Autodesk Inventor part; units mm, degrees
(part 15 of 18)
  ellipse E448 centre (-10.0711, -17.3808) end of major axis (-10.0127, -17.5616) minor radius 0.168 (-10.201, -17.4916) -> (-10.0699, -17.5684) ccw
  ellipse E449 centre (-10.0044, -17.3592) end of major axis (-9.946, -17.54) minor radius 0.168 (-10.1746, -17.347) -> (-10.0032, -17.5468) ccw
  ellipse E450 centre (-10.0405, -11.8092) end of major axis (-10.0989, -11.6284) minor radius 0.168 (-10.0418, -11.6216) -> (-10.2107, -11.797) ccw
  line L564 (-10.1657, -11.65) -> (-10.0989, -11.6284)
  line L565 (-10.0699, -17.5684) -> (-9.8829, -17.5818)
  line L566 (-9.6221, -17.6005) -> (-9.2494, -17.6273)
  line L567 (-10.1746, -17.347) -> (-10.1836, -15.9644)
  line L568 (-9.8264, -17.5595) -> (-10.0032, -17.5468)
  line L569 (-10.0418, -11.6216) -> (-9.5939, -11.6537)
  line L570 (-10.2017, -13.1796) -> (-10.2107, -11.797)
  ellipse E451 centre (-9.5952, -13.6245) end of major axis (-9.6536, -13.4437) minor radius 0.168 (-9.4538, -13.5315) -> (-9.5964, -13.4369) ccw
  ellipse E452 centre (-10.6816, -15.6958) end of major axis (-10.6952, -15.8853) minor radius 0.0836 (-10.7661, -15.7231) -> (-10.7542, -15.813) ccw
  ellipse E453 centre (-10.6948, -13.6615) end of major axis (-10.6812, -13.472) minor radius 0.0836 (-10.696, -13.4739) -> (-10.7106, -13.4814) ccw
  ellipse E454 centre (-10.6948, -13.6615) end of major axis (-10.7084, -13.851) minor radius 0.0836 (-10.7728, -13.6118) -> (-10.7793, -13.6888) ccw
  ellipse E455 centre (-9.5285, -13.603) end of major axis (-9.5869, -13.4222) minor radius 0.168 (-9.4742, -13.4296) -> (-9.5297, -13.4153) ccw
  ellipse E456 centre (-10.5472, -15.7055) end of major axis (-10.5336, -15.516) minor radius 0.0836 (-10.6318, -15.7328) -> (-10.626, -15.7965) ccw
  ellipse E457 centre (-10.5605, -13.6711) end of major axis (-10.5469, -13.4816) minor radius 0.0836 (-10.6385, -13.6213) -> (-10.645, -13.6984) ccw
  line L571 (-10.3369, -13.1699) -> (-10.3459, -11.7873)
  line L572 (-10.4317, -11.627) -> (-10.6574, -11.6999)
  line L573 (-10.7526, -17.6683) -> (-10.3931, -17.5522)
  line L574 (-10.3098, -17.3373) -> (-10.3188, -15.9547)
  line L575 (-10.2026, -13.1795) -> (-10.2116, -11.797)
  line L576 (-10.1755, -17.3469) -> (-10.1845, -15.9644)
  line L577 (-11.2285, -17.875) -> (-10.2588, -17.5619)
  ellipse E458 centre (-10.4305, -11.8146) end of major axis (-10.4169, -11.6251) minor radius 0.0836 (-10.3459, -11.7873) -> (-10.4317, -11.627) ccw
  ellipse E459 centre (-10.3943, -17.3646) end of major axis (-10.4079, -17.5541) minor radius 0.0836 (-10.3931, -17.5522) -> (-10.3098, -17.3373) ccw
  ellipse E460 centre (-10.2961, -11.8243) end of major axis (-10.2825, -11.6347) minor radius 0.0836 (-10.2116, -11.797) -> (-10.2825, -11.6347) ccw
  ellipse E461 centre (-10.26, -17.3742) end of major axis (-10.2736, -17.5637) minor radius 0.0836 (-10.2588, -17.5619) -> (-10.1755, -17.3469) ccw
  line L578 (-10.4169, -11.6251) -> (-10.2825, -11.6347)
  line L579 (-10.9931, -17.9358) -> (-11.1159, -17.927)
  line L580 (-11.1826, -17.9486) -> (-10.9615, -17.9644)
  ellipse E462 centre (-11.0046, -17.8911) end of major axis (-11.2546, -17.8927) minor radius 0.0393 (-11.2285, -17.875) -> (-11.1159, -17.927) ccw
  ellipse E463 centre (-11.0046, -17.8911) end of major axis (-10.6047, -17.8885) minor radius 0.0629 (-11.3596, -17.9224) -> (-11.1826, -17.9486) ccw
  line L581 (9.5691, -13.3926) -> (9.6692, -13.3931)
  line L582 (9.5609, -13.4102) -> (9.5315, -13.41)
  line L583 (9.6942, -15.6278) -> (9.4944, -13.5809)
  ellipse E464 centre (9.7188, -11.8144) end of major axis (9.6943, -11.6259) minor radius 0.0925 (9.7186, -11.6292) -> (9.7004, -11.6256) ccw
  ellipse E465 centre (10.134, -17.4154) end of major axis (10.1585, -17.6038) minor radius 0.0925 (10.1524, -17.6042) -> (10.1585, -17.6038) ccw
  line L584 (10.159, -17.6038) -> (10.1585, -17.6038)
  line L585 (9.7004, -11.6256) -> (9.6471, -11.6253)
  line L586 (9.7129, -17.5843) -> (10.0159, -17.5859)
  line L587 (9.531, -17.601) -> (9.9137, -17.603)
  line L588 (10.1514, -17.6042) -> (10.1524, -17.6042)
  ellipse E466 centre (9.7873, -15.6283) end of major axis (9.8118, -15.8167) minor radius 0.0925 (9.6942, -15.6278) -> (9.7563, -15.7911) ccw
  ellipse E467 centre (9.5875, -13.5814) end of major axis (9.563, -13.393) minor radius 0.0925 (9.5691, -13.3926) -> (9.4944, -13.5809) ccw
  line L589 (-9.3645, -11.6259) -> (-9.6015, -11.6308)
  line L590 (-9.9346, -17.5873) -> (-9.6926, -17.5823)
  line L591 (-9.8266, -17.6047) -> (-9.5717, -17.5995)
  line L592 (-9.6593, -13.3971) -> (-9.5198, -13.3942)
  line L593 (-9.4932, -13.9726) -> (-9.655, -15.6281)
  line L594 (-9.4847, -13.4131) -> (-9.5251, -13.4139)
  ellipse E468 centre (-9.5383, -13.583) end of major axis (-9.5146, -13.3945) minor radius 0.0827 (-9.4531, -13.5262) -> (-9.5198, -13.3942) ccw
  ellipse E469 centre (-9.7384, -15.6298) end of major axis (-9.7147, -15.4413) minor radius 0.0827 (-9.7169, -15.7972) -> (-9.655, -15.6281) ccw
  ellipse E470 centre (-9.2442, -11.6758) end of major axis (-9.6423, -11.6369) minor radius 0.023 (-9.6015, -11.6308) -> (-9.6423, -11.6369) ccw
  line L595 (-9.6423, -11.6369) -> (-9.6436, -11.6502)
  line L596 (11.1852, -17.9034) -> (11.022, -17.917)
  line L597 (11.0263, -17.9438) -> (11.2596, -17.9243)
  ellipse E471 centre (11.1864, -17.7157) end of major axis (11.1349, -17.8986) minor radius 0.1628 (11.1852, -17.9034) -> (11.2728, -17.8675) ccw
  ellipse E472 centre (11.2609, -17.7367) end of major axis (11.2094, -17.9196) minor radius 0.1628 (11.2596, -17.9243) -> (11.3195, -17.9066) ccw
  line L598 (10.4073, -13.401) -> (10.5863, -13.4514)
  line L599 (10.7882, -13.6963) -> (10.7746, -15.7306)
  ellipse E473 centre (10.0601, -13.43) end of major axis (10.4601, -13.4327) minor radius 0.0629 (10.4073, -13.401) -> (9.8616, -13.3741) ccw
  line L600 (9.6609, -13.3908) -> (9.8616, -13.3741)
  line L601 (9.936, -13.3951) -> (9.5169, -13.43)
  ellipse E474 centre (10.0601, -13.43) end of major axis (9.8101, -13.4283) minor radius 0.0393 (10.2771, -13.4119) -> (9.936, -13.3951) ccw
  line L602 (10.4387, -13.4574) -> (10.2771, -13.4119)
  line L603 (9.8455, -15.7837) -> (9.7306, -15.7933)
  ellipse E475 centre (10.044, -15.8396) end of major axis (9.644, -15.8369) minor radius 0.0629 (10.3509, -15.8012) -> (9.8455, -15.7837) ccw
  line L604 (10.6444, -15.7415) -> (10.6474, -15.29)
  line L605 (10.6548, -14.1819) -> (10.658, -13.7071)
  ellipse E476 centre (10.6939, -13.6697) end of major axis (10.6781, -13.4804) minor radius 0.0933 (10.7882, -13.6963) -> (10.7803, -13.6162) ccw
  ellipse E477 centre (10.6804, -15.704) end of major axis (10.6646, -15.5147) minor radius 0.0933 (10.7577, -15.8313) -> (10.7746, -15.7306) ccw
  ellipse E478 centre (10.5637, -13.6806) end of major axis (10.5795, -13.8699) minor radius 0.0933 (10.658, -13.7071) -> (10.6537, -13.6478) ccw
  ellipse E479 centre (10.5501, -15.7149) end of major axis (10.5659, -15.9042) minor radius 0.0933 (10.6441, -15.7534) -> (10.6444, -15.7415) ccw
  ellipse E480 centre (10.5501, -15.7149) end of major axis (10.5659, -15.9042) minor radius 0.0933 (10.6349, -15.8188) -> (10.6426, -15.7751) ccw
  line L606 (10.3796, -17.5684) -> (10.5328, -17.6116)
  line L607 (10.2493, -17.5793) -> (11.3312, -17.8839)
  line L608 (9.8733, -11.6163) -> (9.6559, -11.6344)
  ellipse E481 centre (10.0323, -17.5974) end of major axis (10.2823, -17.5991) minor radius 0.0393 (10.2493, -17.5793) -> (9.9154, -17.5619) ccw
  ellipse E482 centre (10.0718, -11.6722) end of major axis (9.6718, -11.6695) minor radius 0.0629 (10.3988, -11.6381) -> (9.8733, -11.6163) ccw
  ellipse E483 centre (10.0323, -17.5974) end of major axis (9.6323, -17.5947) minor radius 0.0629 (10.3796, -17.5684) -> (9.8379, -17.5412) ccw
  ellipse E484 centre (11.3324, -17.6963) end of major axis (11.3482, -17.8857) minor radius 0.0933 (11.3312, -17.8839) -> (11.3482, -17.8857) ccw
  line L609 (11.4013, -17.8812) -> (11.3482, -17.8857)
  ellipse E485 centre (-10.0243, -17.7521) end of major axis (-10.4666, -17.7632) minor radius 0.0741 (-10.1871, -17.6872) -> (-10.2508, -17.694) ccw
  ellipse E486 centre (-10.174, -17.7137) end of major axis (-10.0241, -17.7099) minor radius 0.0251 (-10.2508, -17.694) -> (-10.312, -17.7072) ccw
  ellipse E487 centre (-10.5584, -17.8746) end of major axis (-10.7084, -17.8783) minor radius 0.0251 (-10.6964, -17.8681) -> (-10.7083, -17.8774) ccw
  ellipse E488 centre (-10.5248, -17.8877) end of major axis (-10.6748, -17.8914) minor radius 0.0251 (-10.6523, -17.904) -> (-10.6494, -17.9047) ccw
  line L610 (-10.6964, -17.8681) -> (-10.6465, -17.8472)
  line L611 (-10.543, -17.8039) -> (-10.5099, -17.79)
  line L612 (-10.3387, -17.7184) -> (-10.312, -17.7072)
  line L613 (-9.0741, -17.7927) -> (-9.1333, -17.8175)
  ellipse E489 centre (-9.8556, -17.818) end of major axis (-9.2758, -17.8034) minor radius 0.0971 (-9.8744, -17.7214) -> (-10.3177, -17.7706) ccw
  ellipse E490 centre (-10.3496, -17.7345) end of major axis (-10.1998, -17.7269) minor radius 0.0268 (-10.3677, -17.7087) -> (-10.3792, -17.7096) ccw
  ellipse E491 centre (-10.3496, -17.7345) end of major axis (-10.1998, -17.7269) minor radius 0.0268 (-10.3138, -17.7067) -> (-10.3238, -17.7068) ccw
  ellipse E492 centre (-10.4338, -17.7442) end of major axis (-10.284, -17.7366) minor radius 0.0268 (-10.5065, -17.7242) -> (-10.5698, -17.7395) ccw
  ellipse E493 centre (-10.8456, -17.924) end of major axis (-10.9954, -17.9315) minor radius 0.0268 (-10.9816, -17.9194) -> (-10.9924, -17.9364) ccw
  ellipse E494 centre (-10.8146, -17.9375) end of major axis (-10.9644, -17.9451) minor radius 0.0268 (-10.9456, -17.957) -> (-10.8774, -17.965) ccw
  line L614 (-10.9961, -17.9176) -> (-10.9954, -17.9315)
  ellipse E495 centre (-10.292, -17.783) end of major axis (-10.734, -17.8053) minor radius 0.0791 (-10.3792, -17.7096) -> (-10.5065, -17.7242) ccw
  ellipse E496 centre (-10.5592, -17.8996) end of major axis (-11.0011, -17.922) minor radius 0.0791 (-10.9924, -17.9364) -> (-10.9456, -17.957) ccw
  line L615 (-10.9816, -17.9194) -> (-10.5698, -17.7395)
  line L616 (-10.646, -17.9728) -> (-10.8774, -17.965)
  ellipse E497 centre (-10.1365, -17.8511) end of major axis (-10.7157, -17.8804) minor radius 0.1037 (-10.1103, -17.7462) -> (-10.6484, -17.9247) ccw
  ellipse E498 centre (10.8498, -17.9277) end of major axis (10.7, -17.9201) minor radius 0.0268 (10.9264, -17.9545) -> (10.9876, -17.945) ccw
  ellipse E499 centre (10.872, -17.9132) end of major axis (11.0218, -17.9208) minor radius 0.0268 (11.0211, -17.9231) -> (11.0008, -17.9058) ccw
  ellipse E500 centre (10.3706, -17.7374) end of major axis (10.5204, -17.745) minor radius 0.0268 (10.4994, -17.73) -> (10.4295, -17.7156) ccw
  ellipse E501 centre (10.2837, -17.7292) end of major axis (10.4335, -17.7368) minor radius 0.0268 (10.2156, -17.7019) -> (10.2072, -17.7023) ccw
  line L617 (11.0218, -17.9208) -> (11.0227, -17.9032)
  ellipse E502 centre (10.5812, -17.894) end of major axis (11.0231, -17.9164) minor radius 0.0791 (10.9876, -17.945) -> (11.0211, -17.9231) ccw
  ellipse E503 centre (10.2559, -17.7799) end of major axis (9.814, -17.7575) minor radius 0.0791 (10.4295, -17.7156) -> (10.3776, -17.7098) ccw
  line L618 (10.4994, -17.73) -> (11.0008, -17.9058)
  line L619 (9.9244, -17.7186) -> (9.9274, -17.7184)
  line L620 (10.1429, -17.706) -> (10.2072, -17.7023)
  line L621 (10.9264, -17.9545) -> (10.6544, -17.9701)
  ellipse E504 centre (10.1447, -17.8527) end of major axis (10.724, -17.882) minor radius 0.1037 (10.6566, -17.9263) -> (10.1185, -17.7477) ccw
  line L622 (9.0199, -17.8982) -> (9.1408, -17.9388)
  ellipse E505 centre (8.5314, -18.0839) end of major axis (9.1087, -18.0281) minor radius 0.1485 (9.1077, -18.0416) -> (9.0262, -17.9624) ccw
  line L623 (-9.1325, -17.937) -> (-9.0106, -17.8853)
  ellipse E506 centre (-8.5232, -18.0826) end of major axis (-9.1005, -18.0268) minor radius 0.1485 (-9.018, -17.961) -> (-9.0995, -18.0402) ccw
  ellipse E507 centre (-9.8417, -17.6845) end of major axis (-9.6917, -17.6835) minor radius 0.0236 (-9.775, -17.663) -> (-9.8671, -17.6614) ccw
  ellipse E508 centre (-9.9269, -17.6896) end of major axis (-9.7769, -17.6886) minor radius 0.0236 (-9.9959, -17.6691) -> (-10.0612, -17.6799) ccw
  ellipse E509 centre (-9.7922, -17.7295) end of major axis (-10.2347, -17.7324) minor radius 0.0696 (-9.8671, -17.6614) -> (-9.9959, -17.6691) ccw
  line L624 (-10.131, -17.7025) -> (-10.0612, -17.6799)
  line L625 (-9.0059, -17.8375) -> (-9.1329, -17.8786)
  line L626 (-9.775, -17.663) -> (-8.9943, -17.719)
  ellipse E510 centre (-9.6485, -17.7958) end of major axis (-9.0685, -17.7921) minor radius 0.0912 (-9.1332, -17.8344) -> (-10.1349, -17.7493) ccw
  ellipse E511 centre (9.1837, -17.6745) end of major axis (9.0344, -17.6891) minor radius 0.0086 (9.3146, -17.666) -> (9.3198, -17.6649) ccw
  ellipse E512 centre (9.1837, -17.6745) end of major axis (9.0344, -17.6891) minor radius 0.0086 (9.2572, -17.6749) -> (9.2595, -17.6746) ccw
  ellipse E513 centre (9.2076, -17.6672) end of major axis (9.3569, -17.6526) minor radius 0.0086 (9.3559, -17.6538) -> (9.3375, -17.6503) ccw
  line L627 (9.3569, -17.6526) -> (9.3542, -17.6252)
  ellipse E514 centre (8.9184, -17.6934) end of major axis (9.3588, -17.6504) minor radius 0.0254 (9.3198, -17.6649) -> (9.3559, -17.6538) ccw
  line L628 (8.9449, -17.6482) -> (9.3375, -17.6503)
  line L629 (9.2572, -17.6749) -> (9.0014, -17.7082)
  ellipse E515 centre (8.4859, -17.7285) end of major axis (9.0632, -17.6721) minor radius 0.0333 (9, -17.6937) -> (8.9426, -17.6636) ccw
  line L630 (-9.3231, -17.6523) -> (-8.937, -17.6444)
  line L631 (-8.9932, -17.7076) -> (-9.2261, -17.6783)
  ellipse E516 centre (-9.1891, -17.6692) end of major axis (-9.3384, -17.6546) minor radius 0.0086 (-9.3231, -17.6523) -> (-9.3362, -17.6564) ccw
  ellipse E517 centre (-9.1603, -17.6769) end of major axis (-9.3096, -17.6623) minor radius 0.0086 (-9.2925, -17.6681) -> (-9.2261, -17.6783) ccw
  line L632 (-9.3367, -17.6373) -> (-9.3384, -17.6546)
  ellipse E518 centre (-8.9024, -17.6942) end of major axis (-9.3428, -17.6512) minor radius 0.0254 (-9.3362, -17.6564) -> (-9.2925, -17.6681) ccw
  ellipse E519 centre (-8.4777, -17.7272) end of major axis (-9.0549, -17.6708) minor radius 0.0333 (-8.9343, -17.6622) -> (-8.9917, -17.6924) ccw
  line L633 (10.0249, -17.6776) -> (10.2019, -17.7274)
  line L634 (10.3294, -17.7633) -> (10.3379, -17.7657)
  line L635 (9.0029, -17.7241) -> (9.7336, -17.6632)
  line L636 (9.1412, -17.8755) -> (9.0142, -17.8398)
  ellipse E520 centre (9.8946, -17.6884) end of major axis (10.0446, -17.6894) minor radius 0.0236 (10.0249, -17.6776) -> (9.9558, -17.6673) ccw
  ellipse E521 centre (9.808, -17.6842) end of major axis (9.958, -17.6852) minor radius 0.0236 (9.8248, -17.6608) -> (9.7336, -17.6632) ccw
  ellipse E522 centre (9.7753, -17.7297) end of major axis (9.3328, -17.7267) minor radius 0.0696 (9.9558, -17.6673) -> (9.8248, -17.6608) ccw
  ellipse E523 centre (9.6567, -17.7973) end of major axis (9.0767, -17.7934) minor radius 0.0912 (10.1432, -17.7508) -> (9.1414, -17.8358) ccw
  line L637 (-10.5777, -15.7864) -> (-10.6036, -15.7973)
  line L638 (-10.6449, -13.7102) -> (-10.63, -13.7039)
  line L639 (-10.5317, -15.7886) -> (-10.5563, -15.7989)
  line L640 (-10.5777, -15.7864) -> (-10.5802, -15.6864)
  ellipse E524 centre (-10.4824, -15.6455) end of major axis (-10.4707, -15.3957) minor radius 0.0974 (-10.4886, -15.3991) -> (-10.5802, -15.6864) ccw
  line L641 (-10.4886, -15.3991) -> (-10.1388, -15.2527)
  line L642 (-10.1021, -15.1377) -> (-10.1321, -13.9452)
  line L643 (-10.1737, -13.863) -> (-10.3951, -13.9557)
  ellipse E525 centre (-10.5297, -13.763) end of major axis (-10.518, -13.5133) minor radius 0.0974 (-10.6275, -13.8039) -> (-10.606, -13.9385) ccw
  line L644 (-10.6275, -13.8039) -> (-10.63, -13.7039)
  line L645 (-10.0861, -13.9473) -> (-10.0561, -15.1399)
  line L646 (-10.584, -13.7061) -> (-10.5815, -13.8061)
  ellipse E526 centre (-10.4837, -13.7652) end of major axis (-10.4954, -14.0149) minor radius 0.0974 (-10.5815, -13.8061) -> (-10.566, -13.9211) ccw
  line L647 (-10.0928, -15.2548) -> (-10.4426, -15.4012)
  ellipse E527 centre (-10.4364, -15.6476) end of major axis (-10.4247, -15.3979) minor radius 0.0974 (-10.4426, -15.4012) -> (-10.5342, -15.6885) ccw
  line L648 (-10.5342, -15.6885) -> (-10.5317, -15.7886)
  line L649 (-10.63, -13.7039) -> (-10.584, -13.7061)
  line L650 (-10.5317, -15.7886) -> (-10.5777, -15.7864)
  ellipse E528 centre (-10.1412, -15.1541) end of major axis (-10.1459, -15.254) minor radius 0.0389 (-10.1388, -15.2527) -> (-10.1021, -15.1377) ccw
  ellipse E529 centre (-10.1712, -13.9616) end of major axis (-10.1665, -13.8617) minor radius 0.0389 (-10.1321, -13.9452) -> (-10.1737, -13.863) ccw
  ellipse E530 centre (-10.0952, -15.1563) end of major axis (-10.0999, -15.2561) minor radius 0.0389 (-10.0928, -15.2548) -> (-10.0561, -15.1399) ccw
  ellipse E531 centre (-10.1252, -13.9637) end of major axis (-10.1205, -13.8638) minor radius 0.0389 (-10.0861, -13.9473) -> (-10.1205, -13.8638) ccw
  line L651 (-10.1665, -13.8617) -> (-10.1205, -13.8638)
  line L652 (9.9214, -15.7283) -> (9.8715, -15.7325)
  line L653 (9.974, -13.6458) -> (9.947, -13.6481)
  line L654 (9.878, -15.7419) -> (9.9486, -15.736)
  ellipse E532 centre (10.132, -15.4618) end of major axis (10.2002, -15.2213) minor radius 0.2063 (9.9291, -15.4231) -> (9.9263, -15.5348) ccw
  ellipse E533 centre (10.1721, -13.878) end of major axis (10.2402, -13.6375) minor radius 0.2063 (9.9691, -13.8393) -> (9.9663, -13.951) ccw
  spline S14 degree 3 poles (10.3544, -15.4547) (10.3538, -15.4489) (10.3525, -15.4373) (10.3493, -15.4202) (10.3452, -15.4035) (10.34, -15.3872) (10.334, -15.3715) (10.3271, -15.3564) (10.3193, -15.3419) (10.3108, -15.3281) (10.3014, -15.3151) (10.2914, -15.3029) (10.2806, -15.2915) (10.2692, -15.2811) (10.2572, -15.2717) (10.2446, -15.2634) (10.2315, -15.2561) (10.2223, -15.2523) (10.2178, -15.2504) knots 0 0 0 0 0.068015 0.135329 0.201939 0.267833 0.332993 0.397396 0.46102 0.523846 0.585863 0.647073 0.70749 0.767154 0.826125 0.884497 0.9424 1 1 1 1
  spline S15 degree 3 poles (10.084, -15.2573) (10.08, -15.2593) (10.072, -15.2634) (10.0606, -15.2705) (10.0495, -15.2783) (10.0389, -15.2869) (10.0288, -15.2961) (10.0192, -15.306) (10.0102, -15.3165) (10.0017, -15.3275) (9.9937, -15.3391) (9.9864, -15.3511) (9.9797, -15.3635) (9.9736, -15.3764) (9.9682, -15.3896) (9.9635, -15.4031) (9.9594, -15.4168) (9.9573, -15.4262) (9.9563, -15.4308) knots 0 0 0 0 0.060188 0.120572 0.181231 0.242221 0.303577 0.365317 0.427444 0.489947 0.552805 0.61599 0.67947 0.743206 0.807162 0.871301 0.93559 1 1 1 1
  spline S16 degree 3 poles (9.9291, -15.4231) (9.9303, -15.4185) (9.9327, -15.4093) (9.9375, -15.3958) (9.9432, -15.3827) (9.9498, -15.3698) (9.9572, -15.3574) (9.9654, -15.3454) (9.9743, -15.3338) (9.9839, -15.3226) (9.9942, -15.312) (10.0051, -15.3019) (10.0165, -15.2923) (10.0284, -15.2833) (10.0408, -15.275) (10.0537, -15.2673) (10.0669, -15.2602) (10.0759, -15.2561) (10.0805, -15.254) knots 0 0 0 0 0.060752 0.121577 0.182585 0.243852 0.305433 0.367353 0.42962 0.492223 0.555134 0.618315 0.681718 0.745286 0.808961 0.872679 0.936378 1 1 1 1
  spline S17 degree 3 poles (10.1858, -15.2319) (10.193, -15.2322) (10.2074, -15.2328) (10.2289, -15.2365) (10.2496, -15.2424) (10.2693, -15.2504) (10.2877, -15.2602) (10.3046, -15.2718) (10.32, -15.285) (10.3341, -15.2996) (10.3468, -15.3155) (10.358, -15.3325) (10.3679, -15.3506) (10.3764, -15.3695) (10.3835, -15.3891) (10.3892, -15.4094) (10.3937, -15.4301) (10.3955, -15.4441) (10.3964, -15.4512) knots 0 0 0 0 0.06487 0.129748 0.194733 0.25818 0.320168 0.381236 0.441837 0.502335 0.563004 0.624034 0.685537 0.747559 0.810091 0.873076 0.936419 1 1 1 1
  spline S18 degree 3 poles (10.3936, -15.5632) (10.3923, -15.5695) (10.3898, -15.5819) (10.384, -15.5996) (10.3768, -15.6164) (10.3681, -15.6321) (10.3581, -15.6467) (10.3467, -15.6602) (10.334, -15.6724) (10.3202, -15.6835) (10.3053, -15.6933) (10.2894, -15.7018) (10.2725, -15.7089) (10.2548, -15.7148) (10.2362, -15.7192) (10.2168, -15.7221) (10.1968, -15.7237) (10.1832, -15.7234) (10.1763, -15.7233) knots 0 0 0 0 0.064651 0.127488 0.188893 0.249239 0.308882 0.368162 0.427398 0.486884 0.546892 0.60767 0.669446 0.732427 0.796802 0.862747 0.930428 1 1 1 1
  spline S19 degree 3 poles (10.0719, -15.7007) (10.0672, -15.6987) (10.0579, -15.6947) (10.0444, -15.6878) (10.0315, -15.6803) (10.0191, -15.6722) (10.0074, -15.6635) (9.9962, -15.6542) (9.9857, -15.6443) (9.976, -15.634) (9.9669, -15.6231) (9.9586, -15.6117) (9.951, -15.5999) (9.9443, -15.5877) (9.9384, -15.575) (9.9334, -15.5619) (9.9293, -15.5485) (9.9273, -15.5394) (9.9263, -15.5348) knots 0 0 0 0 0.066474 0.132184 0.19716 0.261439 0.325059 0.388062 0.450498 0.512425 0.573908 0.635026 0.695866 0.756532 0.81714 0.87782 0.938719 1 1 1 1
  spline S20 degree 3 poles (9.9535, -15.5425) (9.9541, -15.5459) (9.9553, -15.5528) (9.9578, -15.563) (9.9608, -15.5729) (9.9642, -15.5826) (9.9681, -15.5921) (9.974, -15.6044) (9.9823, -15.6191) (9.9939, -15.6358) (10.0069, -15.6513) (10.0211, -15.6658) (10.0315, -15.6744) (10.0367, -15.6787) knots 0 0 0 0 0.064451 0.128324 0.191723 0.254738 0.31745 0.379928 0.504372 0.628458 0.752389 0.876245 1 1 1 1
  spline S21 degree 3 poles (10.251, -15.719) (10.2545, -15.7174) (10.2614, -15.7143) (10.2712, -15.7086) (10.2805, -15.7023) (10.2893, -15.6953) (10.2974, -15.6876) (10.3051, -15.6793) (10.3121, -15.6704) (10.3187, -15.6609) (10.3247, -15.6509) (10.3301, -15.6403) (10.335, -15.6291) (10.3394, -15.6175) (10.3433, -15.6055) (10.3466, -15.593) (10.3495, -15.58) (10.3509, -15.5712) (10.3516, -15.5668) knots 0 0 0 0 0.059947 0.119085 0.177737 0.236204 0.294771 0.353693 0.413202 0.473501 0.534763 0.597137 0.660745 0.725684 0.792031 0.859842 0.929157 1 1 1 1
  spline S22 degree 3 poles (10.3945, -13.8709) (10.3938, -13.8644) (10.3923, -13.8517) (10.3886, -13.8329) (10.3838, -13.8147) (10.3778, -13.797) (10.3707, -13.78) (10.3625, -13.7637) (10.3534, -13.7482) (10.3433, -13.7337) (10.3324, -13.7201) (10.3206, -13.7076) (10.308, -13.6962) (10.2946, -13.686) (10.2806, -13.6772) (10.2659, -13.6697) (10.2507, -13.6636) (10.2401, -13.6609) (10.2348, -13.6595) knots 0 0 0 0 0.068478 0.136179 0.203098 0.269216 0.33451 0.398951 0.462515 0.525184 0.586956 0.647848 0.707903 0.767201 0.825862 0.884056 0.942007 1 1 1 1
  spline S23 degree 3 poles (10.1079, -13.6822) (10.1044, -13.6844) (10.0975, -13.6887) (10.0875, -13.6961) (10.0779, -13.704) (10.0687, -13.7125) (10.0599, -13.7215) (10.0515, -13.7311) (10.0437, -13.7411) (10.0362, -13.7515) (10.0293, -13.7624) (10.0229, -13.7736) (10.017, -13.7852) (10.0117, -13.797) (10.0069, -13.8092) (10.0028, -13.8216) (9.9991, -13.8342) (9.9973, -13.8427) (9.9963, -13.847) knots 0 0 0 0 0.06026 0.120787 0.181623 0.242797 0.30432 0.366196 0.428417 0.490967 0.553825 0.616963 0.680352 0.743961 0.807759 0.871715 0.935803 1 1 1 1
  spline S24 degree 3 poles (9.9691, -13.8393) (9.9702, -13.8351) (9.9725, -13.8265) (9.9768, -13.814) (9.982, -13.8017) (9.9878, -13.7897) (9.9945, -13.778) (10.0018, -13.7667) (10.0097, -13.7558) (10.0183, -13.7452) (10.0275, -13.735) (10.0372, -13.7253) (10.0474, -13.716) (10.0581, -13.7073) (10.0692, -13.699) (10.0808, -13.6913) (10.0926, -13.684) (10.1008, -13.6797) (10.1049, -13.6775) knots 0 0 0 0 0.060837 0.121734 0.182787 0.244069 0.305631 0.367501 0.429693 0.492205 0.555019 0.618108 0.681437 0.744961 0.808632 0.872398 0.936205 1 1 1 1
  spline S25 degree 3 poles (10.2048, -13.6487) (10.2125, -13.6483) (10.2278, -13.6476) (10.2508, -13.6495) (10.2734, -13.6537) (10.2952, -13.6605) (10.3157, -13.6696) (10.3346, -13.6807) (10.3519, -13.6938) (10.3675, -13.7085) (10.3816, -13.7248) (10.3942, -13.7424) (10.4051, -13.7612) (10.4145, -13.781) (10.4224, -13.8017) (10.4287, -13.8231) (10.4335, -13.845) (10.4354, -13.8599) (10.4364, -13.8673) knots 0 0 0 0 0.064914 0.129619 0.19438 0.258975 0.321768 0.383219 0.443897 0.504267 0.56469 0.625418 0.686613 0.748349 0.81063 0.873405 0.936573 1 1 1 1
  spline S26 degree 3 poles (10.4336, -13.9794) (10.4323, -13.986) (10.4296, -13.9991) (10.4234, -14.0178) (10.4155, -14.0353) (10.406, -14.0517) (10.395, -14.0668) (10.3826, -14.0807) (10.3688, -14.0932) (10.3537, -14.1043) (10.3374, -14.114) (10.32, -14.1222) (10.3016, -14.1289) (10.2822, -14.1341) (10.262, -14.1377) (10.241, -14.1396) (10.2193, -14.1399) (10.2047, -14.1388) (10.1972, -14.1381) knots 0 0 0 0 0.064101 0.126323 0.187089 0.246808 0.305872 0.364653 0.423494 0.482714 0.542601 0.60342 0.665411 0.728789 0.793757 0.860499 0.92919 1 1 1 1
  spline S27 degree 3 poles (10.0932, -14.1084) (10.0891, -14.1063) (10.081, -14.1021) (10.0693, -14.095) (10.058, -14.0875) (10.0473, -14.0795) (10.037, -14.071) (10.0274, -14.0621) (10.0183, -14.0527) (10.0098, -14.0428) (10.0019, -14.0326) (9.9947, -14.022) (9.9881, -14.011) (9.9823, -13.9996) (9.9771, -13.9879) (9.9727, -13.9759) (9.969, -13.9636) (9.9672, -13.9552) (9.9663, -13.951) knots 0 0 0 0 0.065853 0.13104 0.19559 0.259537 0.322916 0.38577 0.448145 0.510097 0.571687 0.632987 0.694078 0.755051 0.81601 0.877068 0.938352 1 1 1 1
  spline S28 degree 3 poles (9.9935, -13.9587) (9.9941, -13.9621) (9.9953, -13.969) (9.9978, -13.9791) (10.0008, -13.9891) (10.0042, -13.9988) (10.0082, -14.0083) (10.014, -14.0205) (10.0223, -14.0353) (10.0339, -14.052) (10.0469, -14.0675) (10.0611, -14.082) (10.0715, -14.0905) (10.0768, -14.0948) knots 0 0 0 0 0.064451 0.128324 0.191723 0.254738 0.31745 0.379928 0.504372 0.628458 0.752389 0.876245 1 1 1 1
  spline S29 degree 3 poles (10.2911, -14.1352) (10.2945, -14.1336) (10.3015, -14.1305) (10.3113, -14.1248) (10.3206, -14.1185) (10.3293, -14.1115) (10.3375, -14.1038) (10.3451, -14.0955) (10.3522, -14.0866) (10.3587, -14.0771) (10.3647, -14.067) (10.3702, -14.0564) (10.3751, -14.0453) (10.3795, -14.0337) (10.3833, -14.0217) (10.3866, -14.0091) (10.3895, -13.9962) (10.3909, -13.9874) (10.3916, -13.9829) knots 0 0 0 0 0.059947 0.119085 0.177737 0.236204 0.294771 0.353693 0.413202 0.473501 0.534763 0.597137 0.660745 0.725684 0.792031 0.859842 0.929157 1 1 1 1
  ellipse E534 centre (10.2627, -15.4697) end of major axis (10.2836, -15.7189) minor radius 0.1348 (10.3936, -15.5632) -> (10.3964, -15.4512) ccw
  ellipse E535 centre (10.2208, -15.4732) end of major axis (10.1999, -15.2241) minor radius 0.1348 (10.3516, -15.5668) -> (10.3544, -15.4547) ccw
  ellipse E536 centre (10.3027, -13.8859) end of major axis (10.3236, -14.135) minor radius 0.1348 (10.4336, -13.9794) -> (10.4364, -13.8673) ccw
  ellipse E537 centre (10.2608, -13.8894) end of major axis (10.2399, -13.6403) minor radius 0.1348 (10.3916, -13.9829) -> (10.3945, -13.8709) ccw
  ellipse E538 centre (10.1592, -15.4695) end of major axis (10.0911, -15.7101) minor radius 0.2063 (9.9563, -15.4308) -> (9.9535, -15.5425) ccw
  ellipse E539 centre (10.1992, -13.8857) end of major axis (10.1311, -14.1262) minor radius 0.2063 (9.9963, -13.847) -> (9.9935, -13.9587) ccw
  ellipse E540 centre (10.105, -15.7803) end of major axis (10.3929, -15.7876) minor radius 0.0482 (10.1222, -15.7326) -> (9.9486, -15.736) ccw
  ellipse E541 centre (10.105, -15.7803) end of major axis (10.3929, -15.7876) minor radius 0.0482 (10.3467, -15.7601) -> (10.2191, -15.7389) ccw
  ellipse E542 centre (10.105, -15.7803) end of major axis (9.7671, -15.7718) minor radius 0.0566 (10.3887, -15.7565) -> (10.1782, -15.7269) ccw
  ellipse E543 centre (10.105, -15.7803) end of major axis (9.7671, -15.7718) minor radius 0.0566 (10.0498, -15.7231) -> (9.9214, -15.7283) ccw
  ellipse E544 centre (10.1577, -13.6978) end of major axis (9.8198, -13.6893) minor radius 0.0566 (10.4413, -13.674) -> (10.1781, -13.6418) ccw
  ellipse E545 centre (10.1577, -13.6978) end of major axis (9.8198, -13.6893) minor radius 0.0566 (10.0403, -13.6419) -> (9.974, -13.6458) ccw
  line L655 (10.6007, -15.8166) -> (10.3887, -15.7565)
  line L656 (10.4413, -13.674) -> (10.4721, -13.6827)
  line L657 (10.5601, -13.7077) -> (10.6578, -13.7354)
  line L658 (10.5369, -15.8139) -> (10.3467, -15.7601)
  line L659 (-10.7421, -15.414) -> (-10.4164, -15.2718)
  line L660 (-10.3794, -15.1552) -> (-10.4395, -13.9662)
  line L661 (-10.4863, -13.8862) -> (-10.861, -14.0499)
  ellipse E546 centre (-10.8734, -13.8042) end of major axis (-10.8819, -14.0541) minor radius 0.1052 (-10.9718, -13.9096) -> (-10.861, -14.0499) ccw
  line L662 (-10.3941, -13.9678) -> (-10.3341, -15.1568)
  line L663 (-10.371, -15.2733) -> (-10.6973, -15.4158)
  line L664 (-10.9758, -13.7505) -> (-10.9728, -13.7506)
  ellipse E547 centre (-10.4213, -15.1735) end of major axis (-10.4247, -15.2735) minor radius 0.0421 (-10.4164, -15.2718) -> (-10.3794, -15.1552) ccw
  ellipse E548 centre (-10.4813, -13.9845) end of major axis (-10.478, -13.8846) minor radius 0.0421 (-10.4395, -13.9662) -> (-10.4863, -13.8862) ccw
  ellipse E549 centre (-10.376, -15.175) end of major axis (-10.3794, -15.275) minor radius 0.0421 (-10.371, -15.2733) -> (-10.3341, -15.1568) ccw
  ellipse E550 centre (-10.436, -13.986) end of major axis (-10.4326, -13.8861) minor radius 0.0421 (-10.3941, -13.9678) -> (-10.4326, -13.8861) ccw
  line L665 (-10.478, -13.8846) -> (-10.4326, -13.8861)
  ellipse E551 centre (9.5931, -13.9952) end of major axis (9.5806, -13.8959) minor radius 0.0505 (9.6068, -13.9056) -> (9.5819, -13.8958) ccw
  line L666 (9.5819, -13.8958) -> (9.5255, -13.9001)
  line L667 (10.2287, -15.7604) -> (10.0728, -15.7693)
  line L668 (10.1976, -15.7726) -> (10.2594, -15.769)
  ellipse E552 centre (10.5157, -15.496) end of major axis (10.5984, -15.2601) minor radius 0.2103 (10.3019, -15.5487) -> (10.3038, -15.5637) ccw
  ellipse E553 centre (10.5157, -15.496) end of major axis (10.5984, -15.2601) minor radius 0.2103 (10.3094, -15.4524) -> (10.3038, -15.4807) ccw
  ellipse E554 centre (10.5957, -13.9169) end of major axis (10.6784, -13.681) minor radius 0.2103 (10.3894, -13.8733) -> (10.3838, -13.9846) ccw
  spline S30 degree 3 poles (10.6392, -15.3119) (10.6359, -15.3094) (10.6292, -15.3044) (10.6187, -15.2978) (10.6077, -15.2919) (10.5964, -15.2869) (10.5848, -15.2828) (10.5728, -15.2797) (10.5605, -15.2774) (10.5479, -15.2762) (10.535, -15.276) (10.5219, -15.2769) (10.5086, -15.2789) (10.4952, -15.282) (10.482, -15.2861) (10.4692, -15.2912) (10.4567, -15.2972) (10.4488, -15.3018) (10.4448, -15.3042) knots 0 0 0 0 0.060272 0.120085 0.179563 0.238863 0.298168 0.35769 0.417672 0.478383 0.540118 0.603193 0.66794 0.734231 0.800525 0.866826 0.93328 1 1 1 1
  spline S31 degree 3 poles (10.3497, -15.4169) (10.3482, -15.4205) (10.3452, -15.4277) (10.3413, -15.4387) (10.3378, -15.4499) (10.3359, -15.4575) (10.3349, -15.4613) knots 0 0 0 0 0.249453 0.499322 0.749525 1 1 1 1
  spline S32 degree 3 poles (10.3094, -15.4524) (10.3103, -15.4493) (10.3121, -15.443) (10.3154, -15.4338) (10.319, -15.4248) (10.3231, -15.4159) (10.3276, -15.4072) (10.3325, -15.3987) (10.3378, -15.3903) (10.3416, -15.3849) (10.3435, -15.3822) knots 0 0 0 0 0.124037 0.24816 0.37249 0.497125 0.622143 0.747603 0.873547 1 1 1 1
  spline S33 degree 3 poles (10.4207, -15.3111) (10.4252, -15.3084) (10.4342, -15.303) (10.4482, -15.2958) (10.4626, -15.2893) (10.4772, -15.2837) (10.4921, -15.2789) (10.5071, -15.275) (10.5223, -15.272) (10.5375, -15.2699) (10.5528, -15.2689) (10.5681, -15.2688) (10.5832, -15.2697) (10.5982, -15.2718) (10.6131, -15.275) (10.6275, -15.2793) (10.6415, -15.2846) (10.6504, -15.289) (10.6548, -15.2911) knots 0 0 0 0 0.06406 0.128101 0.192047 0.25583 0.319386 0.382665 0.44563 0.508261 0.570562 0.63256 0.694313 0.755909 0.817476 0.879176 0.940214 1 1 1 1
  spline S34 degree 3 poles (10.6424, -15.749) (10.638, -15.7503) (10.6291, -15.753) (10.6153, -15.756) (10.601, -15.7582) (10.5864, -15.7596) (10.5714, -15.7601) (10.556, -15.7597) (10.5403, -15.7584) (10.5243, -15.7563) (10.508, -15.7532) (10.4916, -15.7493) (10.4754, -15.7444) (10.4596, -15.7388) (10.4443, -15.7323) (10.4296, -15.7251) (10.4154, -15.7172) (10.4064, -15.7113) (10.4019, -15.7084) knots 0 0 0 0 0.054976 0.110963 0.168068 0.226392 0.286031 0.347076 0.409614 0.473728 0.539499 0.606943 0.674365 0.741 0.806864 0.871974 0.936347 1 1 1 1
  spline S35 degree 3 poles (10.3332, -15.6386) (10.3314, -15.6357) (10.3279, -15.63) (10.323, -15.6211) (10.3186, -15.612) (10.3147, -15.6027) (10.3112, -15.5932) (10.3082, -15.5835) (10.3057, -15.5737) (10.3044, -15.567) (10.3038, -15.5637) knots 0 0 0 0 0.125299 0.25024 0.374942 0.499537 0.624172 0.749009 0.874221 1 1 1 1
  spline S36 degree 3 poles (10.3293, -15.5726) (10.3296, -15.5746) (10.3302, -15.5784) (10.3312, -15.5842) (10.3325, -15.5899) (10.3339, -15.5955) (10.3354, -15.6011) (10.3371, -15.6066) (10.339, -15.6121) (10.3404, -15.6156) (10.341, -15.6174) knots 0 0 0 0 0.12683 0.253009 0.378607 0.503687 0.628312 0.752538 0.876418 1 1 1 1
  spline S37 degree 3 poles (10.6235, -15.7576) (10.6252, -15.7568) (10.6287, -15.7554) (10.6337, -15.753) (10.6387, -15.7504) (10.6419, -15.7485) (10.6435, -15.7476) knots 0 0 0 0 0.252829 0.503515 0.752446 1 1 1 1
  spline S38 degree 3 poles (10.6544, -13.7011) (10.6513, -13.7004) (10.645, -13.6991) (10.6354, -13.6978) (10.6257, -13.6971) (10.6158, -13.697) (10.6057, -13.6975) (10.5955, -13.6987) (10.5852, -13.7005) (10.5749, -13.703) (10.5648, -13.7061) (10.5548, -13.7098) (10.5451, -13.714) (10.5356, -13.7188) (10.5263, -13.724) (10.5172, -13.7298) (10.5084, -13.7361) (10.5028, -13.7406) (10.5, -13.7428) knots 0 0 0 0 0.057782 0.11603 0.174905 0.234579 0.295234 0.357058 0.420245 0.484367 0.548389 0.61239 0.67646 0.740675 0.805095 0.869768 0.934728 1 1 1 1
  spline S39 degree 3 poles (10.3894, -13.8733) (10.3897, -13.8722) (10.3903, -13.8699) (10.3913, -13.8666) (10.3923, -13.8633) (10.3931, -13.8611) (10.3935, -13.86) knots 0 0 0 0 0.249966 0.499931 0.749931 1 1 1 1
  spline S40 degree 3 poles (10.4758, -13.7493) (10.4825, -13.7444) (10.4958, -13.7346) (10.5173, -13.722) (10.5396, -13.7112) (10.5628, -13.7025) (10.5864, -13.6958) (10.6065, -13.6921) (10.6226, -13.6904) (10.6347, -13.6898) (10.6467, -13.6897) (10.6547, -13.6902) (10.6587, -13.6904) knots 0 0 0 0 0.126262 0.252787 0.379198 0.50514 0.630313 0.754513 0.81624 0.877714 0.938955 1 1 1 1
  spline S41 degree 3 poles (10.6562, -14.1808) (10.6477, -14.1807) (10.635, -14.1807) (10.6178, -14.179) (10.6047, -14.1772) (10.5913, -14.1748) (10.5733, -14.1707) (10.5512, -14.1642) (10.5257, -14.1541) (10.5016, -14.142) (10.4829, -14.1302) (10.4688, -14.1199) (10.4622, -14.1144) (10.4589, -14.1117) knots 0 0 0 0 0.118368 0.179357 0.241611 0.305185 0.370129 0.500874 0.629162 0.755042 0.878604 0.939568 1 1 1 1
  spline S42 degree 3 poles (10.388, -14.0037) (10.3876, -14.0021) (10.3868, -13.9989) (10.3857, -13.9942) (10.3846, -13.9894) (10.384, -13.9862) (10.3838, -13.9846) knots 0 0 0 0 0.249221 0.498902 0.749131 1 1 1 1
  ellipse E555 centre (10.5412, -15.505) end of major axis (10.4585, -15.7409) minor radius 0.2103 (10.3349, -15.4613) -> (10.3284, -15.4963) ccw
  ellipse E556 centre (10.5412, -15.505) end of major axis (10.4585, -15.7409) minor radius 0.2103 (10.3269, -15.5511) -> (10.3293, -15.5726) ccw
  ellipse E557 centre (10.4664, -15.8171) end of major axis (10.7541, -15.8317) minor radius 0.0515 (10.3606, -15.764) -> (10.321, -15.7655) ccw
  ellipse E558 centre (10.4664, -15.8171) end of major axis (10.7541, -15.8317) minor radius 0.0515 (10.6415, -15.7848) -> (10.4279, -15.7641) ccw
  ellipse E559 centre (10.4664, -15.8171) end of major axis (10.1289, -15.8) minor radius 0.0604 (10.6472, -15.7749) -> (10.3984, -15.7545) ccw
  ellipse E560 centre (10.4664, -15.8171) end of major axis (10.1289, -15.8) minor radius 0.0604 (10.3274, -15.7552) -> (10.2962, -15.7565) ccw
  ellipse E561 centre (10.5716, -13.7408) end of major axis (10.234, -13.7237) minor radius 0.0604 (10.6576, -13.6865) -> (10.4563, -13.6783) ccw
  line L669 (11.6448, -15.7603) -> (11.9491, -15.867)
  line L670 (12.0051, -15.7867) -> (12.0653, -14.5977)
  line L671 (12.0192, -14.4815) -> (11.7149, -14.3748)
  line L672 (11.9062, -15.8695) -> (11.6439, -15.7776)
  ellipse E562 centre (11.9541, -15.7688) end of major axis (11.9598, -15.8686) minor radius 0.051 (11.9491, -15.867) -> (12.0051, -15.7867) ccw
  ellipse E563 centre (12.0143, -14.5798) end of major axis (12.0085, -14.48) minor radius 0.051 (12.0653, -14.5977) -> (12.0192, -14.4815) ccw
  ellipse E564 centre (11.9111, -15.7713) end of major axis (11.9169, -15.8711) minor radius 0.051 (11.9062, -15.8695) -> (11.9169, -15.8711) ccw
  line L673 (11.9598, -15.8686) -> (11.9169, -15.8711)
  line L674 (-10.2822, -15.7509) -> (-10.3285, -15.7659)
  line L675 (-10.462, -13.7179) -> (-10.2958, -13.6642)
  line L676 (-10.2374, -15.7541) -> (-10.2807, -15.7681)
  line L677 (-10.2822, -15.7509) -> (-10.2828, -15.6507)
  ellipse E565 centre (-10.1716, -15.6148) end of major axis (-10.1537, -15.3654) minor radius 0.1101 (-10.1732, -15.3679) -> (-10.2828, -15.6507) ccw
  line L678 (-10.1732, -15.3679) -> (-9.7753, -15.2394)
  line L679 (-9.7314, -15.1262) -> (-9.7392, -13.9313)
  line L680 (-9.7843, -13.8469) -> (-10.0862, -13.9444)
  ellipse E566 centre (-10.1839, -13.7286) end of major axis (-10.166, -13.4792) minor radius 0.1101 (-10.2951, -13.7645) -> (-10.2724, -13.9043) ccw
  line L681 (-10.2951, -13.7645) -> (-10.2958, -13.6642)
  line L682 (-9.6944, -13.9345) -> (-9.6866, -15.1295)
  line L683 (-10.251, -13.6675) -> (-10.2504, -13.7677)
  ellipse E567 centre (-10.1391, -13.7318) end of major axis (-10.157, -13.9811) minor radius 0.1101 (-10.2504, -13.7677) -> (-10.2341, -13.8883) ccw
  line L684 (-9.7305, -15.2426) -> (-10.1285, -15.3711)
  ellipse E568 centre (-10.1269, -15.618) end of major axis (-10.109, -15.3686) minor radius 0.1101 (-10.1285, -15.3711) -> (-10.2381, -15.6539) ccw
  line L685 (-10.2381, -15.6539) -> (-10.2374, -15.7541)
  line L686 (-10.2958, -13.6642) -> (-10.251, -13.6675)
  line L687 (-10.2374, -15.7541) -> (-10.2822, -15.7509)
  ellipse E569 centre (-9.7759, -15.1406) end of major axis (-9.7831, -15.2403) minor radius 0.044 (-9.7753, -15.2394) -> (-9.7314, -15.1262) ccw
  ellipse E570 centre (-9.7837, -13.9457) end of major axis (-9.7765, -13.8459) minor radius 0.044 (-9.7392, -13.9313) -> (-9.7843, -13.8469) ccw
  ellipse E571 centre (-9.7311, -15.1438) end of major axis (-9.7383, -15.2436) minor radius 0.044 (-9.7305, -15.2426) -> (-9.6866, -15.1295) ccw
  ellipse E572 centre (-9.7389, -13.9489) end of major axis (-9.7318, -13.8492) minor radius 0.044 (-9.6944, -13.9345) -> (-9.7318, -13.8492) ccw
  line L688 (-9.7765, -13.8459) -> (-9.7318, -13.8492)
  line L689 (9.7418, -15.7145) -> (9.7139, -15.7169)
  line L690 (9.7557, -13.6279) -> (9.5478, -13.6452)
  line L691 (9.7172, -15.7257) -> (9.7666, -15.7215)
  ellipse E573 centre (9.9549, -15.4471) end of major axis (10.0226, -15.2064) minor radius 0.2142 (9.7438, -15.4088) -> (9.7431, -15.5206) ccw
  ellipse E574 centre (9.9654, -13.8601) end of major axis (10.0332, -13.6195) minor radius 0.2142 (9.7544, -13.8218) -> (9.7537, -13.9337) ccw
  spline S43 degree 3 poles (10.1616, -15.4349) (10.1597, -15.4213) (10.156, -15.3945) (10.1436, -15.3563) (10.1269, -15.3213) (10.1058, -15.2903) (10.0807, -15.264) (10.0521, -15.2432) (10.0256, -15.2312) (10.0033, -15.2253) (9.986, -15.2228) (9.9682, -15.2222) (9.9499, -15.2238) (9.9313, -15.2275) (9.9129, -15.2333) (9.895, -15.2411) (9.8721, -15.2539) (9.8458, -15.274) (9.8184, -15.3037) (9.796, -15.3378) (9.7785, -15.3754) (9.7719, -15.4023) (9.7687, -15.4158) knots 0 0 0 0 0.067054 0.132171 0.195214 0.256087 0.314845 0.371833 0.427831 0.455897 0.484265 0.513193 0.542966 0.573892 0.605563 0.637232 0.669027 0.733247 0.798614 0.865047 0.932273 1 1 1 1
  spline S44 degree 3 poles (9.7438, -15.4088) (9.7456, -15.402) (9.7491, -15.3884) (9.7598, -15.3621) (9.7779, -15.331) (9.8061, -15.2978) (9.8395, -15.2691) (9.877, -15.2457) (9.9175, -15.2281) (9.9597, -15.2173) (9.9956, -15.2144) (10.0239, -15.2164) (10.0447, -15.2201) (10.0647, -15.2259) (10.0836, -15.2338) (10.1012, -15.2435) (10.1226, -15.2586) (10.1462, -15.2816) (10.169, -15.3143) (10.1863, -15.3508) (10.1988, -15.3901) (10.2029, -15.4175) (10.205, -15.4313) knots 0 0 0 0 0.031337 0.062781 0.126297 0.190936 0.256459 0.32232 0.387875 0.452577 0.516183 0.547678 0.57907 0.610325 0.640706 0.670386 0.69965 0.757762 0.816478 0.876441 0.937726 1 1 1 1
  spline S45 degree 3 poles (10.2043, -15.5436) (10.2019, -15.5561) (10.1973, -15.5803) (10.1824, -15.6137) (10.1624, -15.6427) (10.1371, -15.6669) (10.1073, -15.6859) (10.0734, -15.6993) (10.036, -15.707) (9.9955, -15.7086) (9.9529, -15.7038) (9.9101, -15.6929) (9.8695, -15.6759) (9.8328, -15.6535) (9.8009, -15.6263) (9.7788, -15.5999) (9.7644, -15.577) (9.7554, -15.559) (9.748, -15.5402) (9.7447, -15.5272) (9.7431, -15.5206) knots 0 0 0 0 0.060227 0.117303 0.172542 0.227241 0.282631 0.339845 0.399897 0.463695 0.532058 0.603464 0.673189 0.741116 0.807351 0.872143 0.90418 0.93608 0.967968 1 1 1 1
  spline S46 degree 3 poles (9.7679, -15.5276) (9.7686, -15.5309) (9.7699, -15.5375) (9.7725, -15.5472) (9.7755, -15.5567) (9.7802, -15.569) (9.787, -15.584) (9.7969, -15.601) (9.8081, -15.6171) (9.8207, -15.6321) (9.8343, -15.6461) (9.8443, -15.6546) (9.8492, -15.6588) knots 0 0 0 0 0.06406 0.127639 0.190828 0.253706 0.37877 0.503307 0.627605 0.751814 0.875967 1 1 1 1
  spline S47 degree 3 poles (10.0627, -15.7043) (10.0662, -15.7027) (10.0733, -15.6997) (10.0833, -15.694) (10.0926, -15.6877) (10.1014, -15.6805) (10.1095, -15.6727) (10.117, -15.6641) (10.124, -15.655) (10.1303, -15.6451) (10.1361, -15.6347) (10.1413, -15.6237) (10.146, -15.6122) (10.15, -15.6001) (10.1536, -15.5875) (10.1566, -15.5745) (10.1591, -15.561) (10.1603, -15.5519) (10.1609, -15.5472) knots 0 0 0 0 0.059633 0.118254 0.176262 0.234034 0.291919 0.350232 0.409251 0.469215 0.530325 0.592744 0.656603 0.721998 0.789001 0.857656 0.927988 1 1 1 1
  spline S48 degree 3 poles (10.1722, -13.848) (10.1703, -13.8343) (10.1666, -13.8075) (10.1542, -13.7693) (10.1375, -13.7343) (10.1164, -13.7033) (10.0913, -13.677) (10.0627, -13.6562) (10.0362, -13.6442) (10.0139, -13.6383) (9.9966, -13.6358) (9.9788, -13.6352) (9.9604, -13.6368) (9.9419, -13.6405) (9.9234, -13.6463) (9.9056, -13.6541) (9.8827, -13.6669) (9.8564, -13.6871) (9.829, -13.7167) (9.8066, -13.7508) (9.789, -13.7884) (9.7825, -13.8153) (9.7792, -13.8288) knots 0 0 0 0 0.067054 0.132171 0.195214 0.256087 0.314845 0.371833 0.427831 0.455897 0.484265 0.513193 0.542966 0.573892 0.605563 0.637232 0.669027 0.733247 0.798614 0.865047 0.932273 1 1 1 1
  spline S49 degree 3 poles (9.7544, -13.8218) (9.7562, -13.815) (9.7597, -13.8014) (9.7704, -13.7751) (9.7885, -13.7441) (9.8167, -13.7109) (9.8501, -13.6822) (9.8876, -13.6587) (9.9281, -13.6411) (9.9703, -13.6303) (10.0062, -13.6275) (10.0345, -13.6294) (10.0553, -13.6331) (10.0753, -13.6389) (10.0942, -13.6468) (10.1118, -13.6565) (10.1332, -13.6717) (10.1568, -13.6947) (10.1795, -13.7273) (10.1969, -13.7638) (10.2094, -13.8031) (10.2135, -13.8305) (10.2156, -13.8443) knots 0 0 0 0 0.031337 0.062781 0.126297 0.190936 0.256459 0.32232 0.387875 0.452577 0.516183 0.547678 0.57907 0.610325 0.640706 0.670386 0.69965 0.757762 0.816478 0.876441 0.937726 1 1 1 1
  spline S50 degree 3 poles (10.2148, -13.9567) (10.2125, -13.9691) (10.2079, -13.9934) (10.193, -14.0267) (10.1729, -14.0557) (10.1477, -14.0799) (10.1179, -14.0989) (10.084, -14.1124) (10.0466, -14.12) (10.0061, -14.1216) (9.9635, -14.1168) (9.9207, -14.1059) (9.8801, -14.0889) (9.8434, -14.0665) (9.8115, -14.0393) (9.7894, -14.0129) (9.775, -13.99) (9.766, -13.972) (9.7586, -13.9532) (9.7553, -13.9402) (9.7537, -13.9337) knots 0 0 0 0 0.060227 0.117303 0.172542 0.227241 0.282631 0.339845 0.399897 0.463695 0.532058 0.603464 0.673189 0.741116 0.807351 0.872143 0.90418 0.93608 0.967968 1 1 1 1
  spline S51 degree 3 poles (9.7785, -13.9406) (9.7792, -13.9439) (9.7805, -13.9505) (9.7831, -13.9602) (9.7861, -13.9697) (9.7908, -13.982) (9.7976, -13.997) (9.8074, -14.014) (9.8187, -14.0301) (9.8312, -14.0451) (9.8449, -14.0592) (9.8548, -14.0676) (9.8598, -14.0718) knots 0 0 0 0 0.06406 0.127639 0.190828 0.253706 0.37877 0.503307 0.627605 0.751814 0.875967 1 1 1 1
  spline S52 degree 3 poles (10.0733, -14.1173) (10.0768, -14.1158) (10.0839, -14.1127) (10.0938, -14.107) (10.1032, -14.1007) (10.1119, -14.0935) (10.1201, -14.0857) (10.1276, -14.0772) (10.1346, -14.068) (10.1409, -14.0582) (10.1467, -14.0477) (10.1519, -14.0367) (10.1565, -14.0252) (10.1606, -14.0131) (10.1642, -14.0006) (10.1671, -13.9875) (10.1696, -13.9741) (10.1708, -13.9649) (10.1714, -13.9603) knots 0 0 0 0 0.059633 0.118254 0.176262 0.234034 0.291919 0.350232 0.409251 0.469215 0.530325 0.592744 0.656603 0.721998 0.789001 0.857656 0.927988 1 1 1 1
  ellipse E575 centre (10.0838, -15.4534) end of major axis (10.1046, -15.7026) minor radius 0.1227 (10.2043, -15.5436) -> (10.205, -15.4313) ccw
  ellipse E576 centre (10.0404, -15.4571) end of major axis (10.0197, -15.2079) minor radius 0.1227 (10.1609, -15.5472) -> (10.1616, -15.4349) ccw
  ellipse E577 centre (10.0944, -13.8665) end of major axis (10.1152, -14.1156) minor radius 0.1227 (10.2148, -13.9567) -> (10.2156, -13.8443) ccw
  ellipse E578 centre (10.051, -13.8701) end of major axis (10.0302, -13.621) minor radius 0.1227 (10.1714, -13.9603) -> (10.1722, -13.848) ccw
  ellipse E579 centre (9.9797, -15.4541) end of major axis (9.9119, -15.6947) minor radius 0.2142 (9.7687, -15.4158) -> (9.7679, -15.5276) ccw
  ellipse E580 centre (9.9903, -13.8671) end of major axis (9.9225, -14.1077) minor radius 0.2142 (9.7792, -13.8288) -> (9.7785, -13.9406) ccw
  ellipse E581 centre (9.9095, -15.7618) end of major axis (10.1975, -15.7637) minor radius 0.0453 (10.1596, -15.7409) -> (9.7666, -15.7215) ccw
  ellipse E582 centre (9.9095, -15.7618) end of major axis (9.5715, -15.7595) minor radius 0.0531 (10.203, -15.7373) -> (9.7418, -15.7145) ccw
  ellipse E583 centre (9.9234, -13.6751) end of major axis (9.5855, -13.6729) minor radius 0.0531 (10.2169, -13.6506) -> (9.7557, -13.6279) ccw
  line L692 (10.3622, -15.7821) -> (10.203, -15.7373)
  line L693 (10.2169, -13.6506) -> (10.2335, -13.6553)
  line L694 (10.2492, -13.6598) -> (10.2621, -13.6634)
  line L695 (10.3201, -15.7862) -> (10.1596, -15.7409)
  line L696 (-10.5562, -13.6815) -> (-10.4497, -13.6865)
  ellipse E584 centre (10.4637, -13.3559) end of major axis (10.3792, -13.6542) minor radius 0.2558 (10.456, -13.6615) -> (10.4698, -13.6599) ccw
  line L697 (10.4698, -13.6599) -> (10.5371, -13.6789)
  line L698 (10.4064, -13.6656) -> (10.456, -13.6615)
  arc A6 (-11.8168, -13.8235) -> (-11.7156, -13.9335) centre (-11.5448, -13.6748) ccw
  ellipse E585 centre (10.4587, -13.7718) end of major axis (10.9007, -13.7942) minor radius 0.0791 (10.658, -13.7109) -> (10.6459, -13.7092) ccw
  arc A7 (11.7375, -13.9301) -> (11.8628, -13.8077) centre (11.5924, -13.6561) ccw
  ellipse E586 centre (-10.2656, -13.3341) end of major axis (-10.1703, -13.6291) minor radius 0.274 (-10.2784, -13.6388) -> (-10.2636, -13.6402) ccw
  line L699 (-10.2938, -13.6437) -> (-10.2784, -13.6388)
  line L700 (-10.2636, -13.6402) -> (-10.1241, -13.6503)
  ellipse E587 centre (9.6613, -13.3025) end of major axis (9.687, -13.6114) minor radius 0.1522 (9.6506, -13.6057) -> (9.6592, -13.6086) ccw
  line L701 (9.5508, -13.614) -> (9.6506, -13.6057)
  ellipse E588 centre (10.225, -13.3302) end of major axis (10.1409, -13.6286) minor radius 0.2656 (10.2229, -13.6363) -> (10.2372, -13.6347) ccw
  line L702 (10.2372, -13.6347) -> (10.2871, -13.6487)
  line L703 (10.1714, -13.6406) -> (10.2229, -13.6363)
  line L704 (9.6592, -13.6086) -> (9.712, -13.6235)
  ellipse E589 centre (9.802, -13.7016) end of major axis (10.2445, -13.7045) minor radius 0.0696 (10.0222, -13.6426) -> (9.9961, -13.6403) ccw
  arc A8 (-10.3559, -15.7646) -> (-10.4901, -15.7883) centre (-10.3704, -16.0742) ccw
  line L705 (-10.4901, -15.7883) -> (-10.5359, -15.8074)
  line L706 (-10.0301, -15.7798) -> (-10.3559, -15.7646)
  arc A9 (-10.7625, -15.8155) -> (-10.7777, -15.8217) centre (-10.6536, -16.1058) ccw
  arc A10 (-10.6431, -15.7959) -> (-10.7345, -15.8065) centre (-10.6536, -16.1058) ccw
  line L707 (-10.7777, -15.8217) -> (-10.8679, -15.8611)
  line L708 (-10.5185, -15.8002) -> (-10.6431, -15.7959)
  arc A11 (-9.3975, -21.1651) -> (-9.3954, -21.1643) centre (-9.7999, -20.0346) ccw
  line L709 (9.1866, -20.2306) -> (9.2854, -21.1744)
  line L710 (-9.1787, -20.2292) -> (-9.2777, -21.173)
  arc A12 (9.4032, -21.1658) -> (9.4053, -21.1665) centre (9.8078, -20.0361) ccw
  arc A13 (6.4067, -24.0066) -> (6.5223, -23.981) centre (6.2058, -22.8235) ccw
  line L711 (6.7093, -22.7152) -> (6.7222, -22.7735)
  arc A14 (-6.515, -23.98) -> (-6.3994, -24.0056) centre (-6.1983, -22.8226) ccw
  line L712 (-6.7018, -22.7142) -> (-6.7146, -22.7725)
  arc A15 (-10.2624, -22.9884) -> (-9.7725, -23.0227) centre (-9.9354, -21.8338) ccw
  line L713 (-11.0301, -10.3637) -> (-11.0206, -10.5511)
  line L714 (-10.969, -11.5733) -> (-10.9618, -11.716)
  line L715 (-10.6517, -17.8603) -> (-10.5348, -20.1748)
  line L716 (-10.4805, -21.2507) -> (-10.4461, -21.9322)
  arc A16 (-7.3485, -23.8906) -> (-7.2302, -23.8968) centre (-7.2264, -22.6968) ccw
  line L717 (-6.7114, -22.7112) -> (-6.7146, -22.7725)
  line L718 (-7.7007, -21.9108) -> (-7.7511, -22.8672)
  line L719 (5.5117, -21.7652) -> (5.5279, -21.842)
  arc A17 (8.8957, -24.2113) -> (9.1947, -24.1776) centre (8.9119, -23.0114) ccw
  line L720 (9.3383, -22.1971) -> (9.4444, -23.1378)
  line L721 (8.3139, -22.3043) -> (8.4208, -23.2531)
  arc A18 (-9.1874, -24.1762) -> (-8.8884, -24.21) centre (-8.9044, -23.0101) ccw
  line L722 (-8.3063, -22.303) -> (-8.4134, -23.2518)
  line L723 (-9.3307, -22.1956) -> (-9.4369, -23.1363)